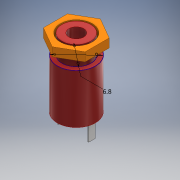
# Autodesk Inventor part: headphone jack
Saved by Autodesk Inventor 2018 (Build 220112000, 112)
## iProperties
Created: 2017-12-11
Part Number: headphone jack
Material: Generic
Document SubType Name: Modeling
Designer: caleb
Density: 1 g/cm^3
Appearance: Default
Author: caleb
Autodesk Inventor part; units mm, degrees
ref_plane "YZ Plane" through (0, 0, 0) normal (1, 0, 0) x (0, 1, 0)
ref_plane "XZ Plane" through (0, 0, 0) normal (0, 1, 0) x (-1, 0, 0)
ref_plane "XY Plane" through (0, 0, 0) normal (0, 0, 1) x (1, 0, 0)
sketch "Sketch1" plane through (0, 0, 0) normal (0, 0, 1) x (1, 0, 0)
  circle A0 centre (0, 0) radius 4.5
  circle A1 centre (0, 0) radius 3.4
  dimension "d0" = 9
  dimension "d1" = 6.8
  constraints: 2 centre point, 2 coincident
  measures "d0" diameter of A0
  measures "d1" diameter of A1
extrude "Extrusion1" add sketch "Sketch1" against normal blind 11.684 contours A0 | A1
extrude "Extrusion2" add sketch "Sketch1" along normal blind 4.4958 contours A1
sketch "Sketch2" plane through (0, 0, 4.4958) normal (0, 0, 1) x (1, 0, 0)
  circle A0 centre (0, 0) radius 1.75
  dimension "d6" = 3.5
  constraints: 1 centre point, 1 coincident
  measures "d6" diameter of A0
extrude "Extrusion3" cut sketch "Sketch2" against normal blind 21.4958
sketch "Sketch3" plane through (0, 0, 4.4958) normal (0, 0, 1) x (1, 0, 0)
  line L0 (4.9213, -2.8413) -> (0, -5.6826)
  line L1 (0, -5.6826) -> (-4.9213, -2.8413)
  line L2 (-4.9213, -2.8413) -> (-4.9213, 2.8413)
  line L3 (-4.9213, 2.8413) -> (0, 5.6826)
  line L4 (0, 5.6826) -> (4.9212, 2.8413)
  line L5 (4.9212, 2.8413) -> (4.9213, -2.8413)
  circle A0 centre (0, 0) radius 3.7725
  dimension "d9" = 9.8425
  dimension "d12" = 7.5451
  constraints: 12 end point, 2 coincident, 1 centre point, 1 vertical, 13 other
  measures "d9" distance between parallel lines of L4 L1
  measures "d12" diameter of A0
extrude "Extrusion4" add sketch "Sketch3" against normal blind 2.0574 separate body
sketch "Sketch4" plane through (0, 0, -11.684) normal (0, 0, -1) x (-1, 0, 0)
  line L0 (-3.6931, -0.77) -> (-3.4931, -0.77)
  line L1 (-3.4931, -0.77) -> (-3.4931, 0.77)
  line L2 (-3.4931, 0.77) -> (-3.6931, 0.77)
  line L3 (-3.6931, 0.77) -> (-3.6931, -0.77)
  circle A0 centre (0, 0) radius 3.7725 projected
  line L4 (-0.77, 3.4931) -> (0.77, 3.4931)
  line L5 (0.77, 3.4931) -> (0.77, 3.6931)
  line L6 (0.77, 3.6931) -> (-0.77, 3.6931)
  line L7 (-0.77, 3.6931) -> (-0.77, 3.4931)
  line L8 (3.4931, -0.77) -> (3.6931, -0.77)
  line L9 (3.6931, -0.77) -> (3.6931, 0.77)
  line L10 (3.6931, 0.77) -> (3.4931, 0.77)
  line L11 (3.4931, 0.77) -> (3.4931, -0.77)
  point P0 (3.4931, 0)
  point P1 (-3.4931, 0)
  dimension "d13" = 0.2
  dimension "d14" = 1.54
  constraints: 24 end point, 6 parallel, 6 point on circle, 4 equal length, 3 horizontal, 3 perpendicular, 2 horizontal alignment, 2 midpoint
  measures "d13" distance of L1.end L2.end
  measures "d14" distance of L0.end L1.end
extrude "Extrusion5" add sketch "Sketch4" along normal blind 3.9624 separate body contours L3 L2 L1 L0 | L8 L11 L10 L9 | L6 L5 L4 L7
body "Solid1"
body "Solid2"
body "Solid3"
